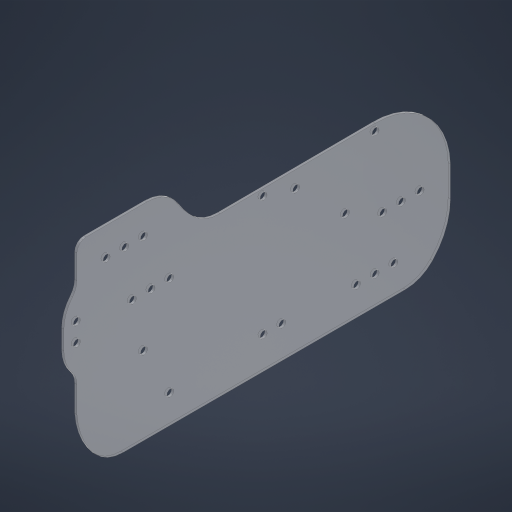
# Autodesk Inventor part: dtplate2
Saved by Autodesk Inventor 2024 (Build 280153000, 153)
## iProperties
Created: 2023-11-04
Part Number: dtplate2
Material: Generic
Document SubType Name: Modeling
Designer: macbook
Density: 1 g/cm^3
Appearance: Polycarbonate - Clear
Author: macbook
Autodesk Inventor part; units mm, degrees
ref_plane "YZ Plane" through (0, 0, 0) normal (1, 0, 0) x (0, 1, 0)
ref_plane "XZ Plane" through (0, 0, 0) normal (0, 1, 0) x (-1, 0, 0)
ref_plane "XY Plane" through (0, 0, 0) normal (0, 0, 1) x (1, 0, 0)
sketch "Sketch1" plane through (0, 0, 0) normal (1, 0, 0) x (0, 1, 0)
  line L0 (-0.08, -0.0424) -> (33.575, -0.0424) construction
  line L1 (-0.08, -0.0424) -> (33.575, 17.8168) construction
  line L2 (33.575, 17.8168) -> (67.23, 17.8168) construction
  line L3 (67.2525, 0) -> (100.9075, 17.8592) construction
  line L4 (67.2525, 0) -> (67.2525, 12.7) construction
  line L5 (67.2525, 12.7) -> (67.2525, 25.4) construction
  line L6 (100.9075, 17.8592) -> (100.9075, 30.5592) construction
  line L7 (100.9075, 30.5592) -> (100.9075, 43.2592) construction
  line L8 (-0.08, -0.0424) -> (-0.08, -25.4424) construction
  line L9 (-0.08, -25.4424) -> (-0.08, -50.8424) construction
  line L10 (-0.08, -88.9424) -> (-0.08, -127.0424) construction
  line L11 (-0.08, -127.0424) -> (-0.08, -139.7424) construction
  line L12 (-0.08, -139.7424) -> (-0.08, -152.4424) construction
  line L13 (-0.08, -127.0424) -> (33.575, -127.0424) construction
  line L14 (-0.08, -127.0424) -> (33.575, -144.9016) construction
  line L15 (33.575, -144.9016) -> (33.575, -157.6016) construction
  line L16 (33.575, -157.6016) -> (33.575, -170.3016) construction
  line L17 (33.575, 17.8168) -> (67.23, -0.0424) construction
  line L18 (67.2525, 25.4) -> (67.2525, 63.5) construction
  line L19 (67.2525, 63.5) -> (73.6025, 63.5) construction
  line L20 (67.2525, 63.5) -> (60.9025, 63.5) construction
  line L21 (-0.08, -0.0424) -> (-19.13, -0.0424)
  line L22 (-19.13, -0.0424) -> (-19.13, 32.0447)
  line L23 (-19.13, -0.0424) -> (-19.13, -160.046)
  line L24 (36.697, 63.4964) -> (-19.13, 63.4576)
  line L25 (97.8052, 63.5389) -> (114.0388, 63.5502)
  line L26 (82.2933, 63.5281) -> (82.3639, -38.0718)
  line L27 (-19.13, -190.5424) -> (18.97, -190.5424)
  line L28 (-19.13, 63.4576) -> (18.97, 63.4841)
  line L29 (-19.13, -190.5424) -> (-19.13, -168.3174)
  line L30 (-19.13, 63.4576) -> (-19.13, 41.2326)
  arc A0 (-11.2913, -178.3971) -> (18.97, -190.5424) centre (18.9669, -146.7782) ccw
  arc A1 (18.97, 63.4841) -> (-10.529, 51.096) centre (22.5987, 13.5269) ccw
  arc A2 (-10.529, 51.096) -> (-19.13, 32.0447) centre (6.27, 32.0447) ccw
  arc A3 (-19.13, -160.046) -> (-11.2913, -178.3971) centre (6.27, -160.046) ccw
  line L31 (18.97, -190.5424) -> (39.8188, -190.5569)
  line L32 (82.47, -190.5424) -> (82.4192, -117.5175)
  arc A4 (59.3801, -181.3807) -> (82.4192, -117.5175) centre (-17.5044, -117.5566) ccw
  arc A5 (39.8188, -190.5569) -> (59.3801, -181.3807) centre (39.8365, -165.157) ccw
  line L33 (120.3932, 57.2002) -> (120.3932, 15.8527)
  arc A6 (108.3748, -5.7365) -> (95.266, -16.5881) centre (141.2935, -58.8459) ccw
  arc A7 (108.3748, -5.7365) -> (120.3932, 15.8527) centre (94.9932, 15.8527) ccw
  arc A8 (84.8043, -32.1396) -> (82.3674, -43.0135) centre (107.7674, -42.9958) ccw
  arc A9 (120.3932, 57.2002) -> (114.0388, 63.5502) centre (114.0432, 57.2002) ccw
  line L34 (60.9025, 63.5) -> (52.0125, 63.5071)
  line L35 (60.9025, 63.5) -> (60.9025, 72.39)
  line L36 (60.9025, 72.39) -> (73.66, 72.39)
  line L37 (73.6025, 63.5) -> (86.3025, 63.5309) construction
  line L38 (60.9025, 63.5) -> (41.8525, 63.5)
  line L39 (41.8525, 63.5) -> (73.6025, 63.5)
  line L40 (73.6025, 63.5) -> (92.6525, 63.5353)
  arc A10 (89.6573, 66.4898) -> (73.66, 72.39) centre (73.3791, 46.9916) ccw
  arc A11 (60.9025, 72.39) -> (44.8441, 66.4614) centre (61.1559, 46.9913) ccw
  arc A12 (89.6573, 66.4898) -> (97.8052, 63.5389) centre (97.7963, 76.2389) ccw
  arc A13 (36.697, 63.4964) -> (44.8441, 66.4614) centre (36.6882, 76.1964) ccw
  line L41 (82.3639, -38.0718) -> (82.3816, -63.4718)
  line L42 (82.3816, -63.4718) -> (88.7316, -63.4718)
  line L43 (88.7316, -63.4718) -> (88.5767, -33.8992)
  line L44 (82.3816, -63.4718) -> (83.9691, -63.4718)
  line L45 (83.9691, -63.4718) -> (83.9691, -139.6718)
  line L46 (88.7316, -63.4718) -> (89.1289, -139.2994)
  arc A14 (95.266, -16.5881) -> (88.5767, -33.8992) centre (113.9763, -33.7661) ccw
  arc A15 (36.6882, -190.5548) -> (89.1289, -139.2994) centre (38.1214, -139.5667) ccw
  line L47 (2.4584, -63.5424) -> (2.4584, -76.2424)
  line L48 (2.4584, -63.5424) -> (-0.0816, -63.5424)
  line L49 (-0.08, -50.8424) -> (-0.08, -88.9424)
  line L50 (82.3816, -63.4718) -> (77.3016, -63.4718)
  line L51 (77.3016, -63.4718) -> (77.3016, -85.6968)
  line L52 (83.9691, -139.6718) -> (45.6151, -139.6718)
  line L53 (45.6151, -139.6718) -> (45.6151, -119.5296)
  point P0 (120.3932, 63.5546)
  point P1 (50.72, -190.5645)
  point P2 (120.3932, 0.039)
  point P3 (50.7001, 63.5062)
  point P4 (88.532, -25.3724)
  point P5 (82.2933, 63.5161)
  point P6 (82.2933, 63.5212)
  point P7 (39.4835, -190.5567)
  point P8 (79.9412, -139.6718)
  point P9 (82.4346, -139.6718)
  dimension "d81" = 33.655
  dimension "d82" = 38.1
  dimension "d83" = 33.655
  dimension "d84" = 38.1
  dimension "d85" = 38.1
  dimension "d88" = 12.7
  dimension "d89" = 12.7
  dimension "d90" = 12.7
  dimension "d91" = 12.7
  dimension "d92" = 25.4
  dimension "d93" = 25.4
  dimension "d94" = 38.1
  dimension "d95" = 38.1
  dimension "d96" = 12.7
  dimension "d97" = 12.7
  dimension "d98" = 33.655
  dimension "d99" = 38.1
  dimension "d100" = 12.7
  dimension "d101" = 12.7
  dimension "d109" = 38.1
  dimension "d110" = 38.1
  dimension "d111" = 6.35
  dimension "d112" = 6.35
  dimension "d122" = 19.05
  dimension "d123" = 63.5
  dimension "d124" = 190.5
  dimension "d125" = 101.6
  dimension "d126" = 38.1
  dimension "d127" = 101.6
  dimension "d128" = 38.1
  dimension "d129" = 38.1
  dimension "d130" = 22.225
  dimension "d131" = 22.225
  dimension "d132" = 43.7642
  dimension "d133" = 50.0888
  dimension "d134" = 25.4
  dimension "d135" = 31.75
  dimension "d136" = 73.025
  dimension "d137" = 99.9236
  dimension "d138" = 25.4
  dimension "d139" = 62.484
  dimension "d140" = 25.4
  dimension "d141" = 6.35
  dimension "d142" = 8.89
  dimension "d143" = 8.89
  dimension "d144" = 12.7
  dimension "d145" = 19.05
  dimension "d146" = 19.05
  dimension "d147" = 25.4
  dimension "d148" = 25.4
  dimension "d149" = 12.7
  dimension "d150" = 25.4
  dimension "d151" = 6.35
  dimension "d152" = 38.1
  dimension "d153" = 1.5875
  dimension "d154" = 76.2
  dimension "d155" = 25.4
  dimension "d159" = 2.54
  dimension "d160" = 5.08
  dimension "d161" = 22.225
  dimension "d162" = 38.354
  dimension "d163" = 20.1422
  constraints: 108 end point, 41 point on circle, 25 point on line, 21 coincident, 18 tangent, 16 centre point, 13 vertical, 10 horizontal, 4 perpendicular, 3 equal radius, 1 collinear, 1 other
  measures "d81" distance of L0.start L0.end
  measures "d82" distance of L0.start L1.end
  measures "d83" distance of L1.end L2.end
  measures "d84" distance of L1.end L3.start
  measures "d85" distance of L3.start L3.end
  measures "d88" distance of L3.start L4.end
  measures "d89" distance of L4.end L5.end
  measures "d90" distance of L3.end L6.end
  measures "d91" distance of L6.end L7.end
  measures "d92" distance of L0.start L8.end
  measures "d93" distance of L8.end L9.end
  measures "d94" distance of L9.end L10.start
  measures "d95" distance of L10.start L10.end
  measures "d96" distance of L10.end L11.end
  measures "d97" distance of L11.end L12.end
  measures "d98" distance of L13.start L13.end
  measures "d99" distance of L13.start L14.end
  measures "d100" distance of L15.start L15.end
  measures "d101" distance of L15.end L16.end
  measures "d109" distance of L17.start L17.end
  measures "d110" distance of L18.start L18.end
  measures "d111" distance of L18.end L19.end
  measures "d112" distance of L18.end L20.end
  measures "d122" distance of L0.start L21.end
  measures "d123" distance of L21.end L24.end
  measures "d124" distance of L21.end L27.start
  measures "d125" distance of L27.start L32.start
  measures "d126" distance of L26.start point (120.393, 63.555)
  measures "d127" distance of L26.start L26.end
  measures "d128" distance of L27.start L27.end
  measures "d129" distance of L24.end L28.end
  measures "d130" distance of L27.start L29.end
  measures "d131" distance of L24.end L30.end
  measures "d132" radius of A0
  measures "d133" radius of A1
  measures "d134" radius of A2
  measures "d135" distance of L27.end point (50.72, -190.565)
  measures "d136" distance of L32.start L32.end
  measures "d137" radius of A4
  measures "d138" radius of A5
  measures "d139" radius of A6
  measures "d140" radius of A7
  measures "d141" radius of A9
  measures "d142" distance of L34.start L34.end
  measures "d143" distance of L34.start L35.end
  measures "d144" distance of L37.start L37.end
  measures "d145" distance of L34.start L38.end
  measures "d146" distance of L37.start L40.end
  measures "d147" radius of A10
  measures "d148" radius of A11
  measures "d149" radius of A12
  measures "d150" distance of L26.end L41.end
  measures "d151" distance of L41.end L42.end
  measures "d152" distance of L42.end point (88.532, -25.372)
  measures "d153" distance of L41.end L44.end
  measures "d154" distance of L44.end L45.end
  measures "d155" radius of A14
  measures "d159" distance of L47.start L48.end
  measures "d160" distance of L41.end L50.end
  measures "d161" distance of L50.end L51.end
  measures "d162" distance of L52.start L52.end
  measures "d163" distance of L52.end L53.end
extrude "Extrusion1" add sketch "Sketch1" along normal blind 1.5875 contours L22 A2 A1 L24 A13 A11 L35 L39 L40 L26 L41 L42 L45 L52 L32 A4 A5 A15 L31 A0 A3 L23 | L36 A10 A12 L25 A9 L33 A7 A6 A14 L43 L42 L41 L26 L40 L39 L35 | A5 A4 L52 L32 A15 | L32 L52 L45 L42 L46 A15 | A4 L32 L52
hole "Hole4" at (0, -0.08, -0.0424) at (0, -0.08, -127.0424) at (0, -0.08, -139.7424) at (0, -0.08, -152.4424) at (0, 33.575, -144.9016) at (0, 100.9075, 43.2592) at (0, 100.9075, 30.5592) at (0, 100.9075, 17.8592) at (0, 67.2525, 25.4) at (0, 67.2525, 12.7) at (0, 67.2525, 0) at (0, 33.575, 17.8168) at (0, 33.575, -157.6016) at (0, 33.575, -170.3016) at (0, 73.6025, 63.5) at (0, 60.9025, 63.5) at (0, 2.4584, -63.5424) at (0, 2.4584, -76.2424) at (0, 83.9691, -63.4718) at (0, 83.9691, -139.6718) at (0, 45.6151, -119.5296) at (0, 77.3016, -85.6968) direction (1, 0, 0) diameter 4.7625 end through all
body "Solid1"
